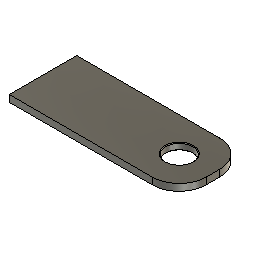
Lasche_19 (Autodesk Fusion 360 design; units mm, degrees)
Autodesk Fusion 360 part; units mm, degrees
sketch "Sketch1" plane through (0, 0, 0) normal (0, 0, 1) x (1, 0, 0)
  line L0 (-20.19, -5) -> (0, -5)
  line L1 (0, -5) -> (0, 5)
  line L2 (0, 5) -> (-20.19, 5)
  line L3 (-20.19, 5) -> (-20.19, -5)
  line L4 (0, 5) -> (1, 5)
  line L5 (5, 1) -> (5, -1)
  line L6 (1, -5) -> (0, -5)
  line L7 (0, -5) -> (0, 5)
  arc A0 (1, -5) -> (5, -1) centre (1, -1) ccw
  arc A1 (5, 1) -> (1, 5) centre (1, 1) ccw
  circle A2 centre (0, 0) radius 2
  point P0 (5, 5)
  dimension "d1" = 20.19
  dimension "d2" = 10
  dimension "d3" = 5
  dimension "d5" = 4
  dimension "d6" = 4
  dimension "d7" = 4
  constraint horizontal L0
  constraint vertical L1
  constraint horizontal L2
  constraint vertical L3
  constraint horizontal L4
  constraint vertical L5
  constraint horizontal L6
  constraint vertical L7
  constraint tangent L5 A0
  constraint tangent L6 A0
  constraint coincident P0 L4
  constraint coincident P0 L5
  constraint tangent L4 A1
  constraint tangent L5 A1
  constraint midpoint L1 A2.centre
  constraint coincident A2.centre origin
  measures "d1" distance of L0.start L0.end
  measures "d2" distance of L0.start L2.end
  measures "d3" distance of L1.end P0
  measures "d5" radius of A0
  measures "d6" radius of A1
  measures "d7" diameter of A2
extrude "Extrude1" add sketch "Sketch1" along normal mid plane 1 contours L0 L1 L2 L3 L7 A2 | L1 L4 L5 L6 L7 A0 A1 A2
chamfer "Chamfer1" distance 0.1 angle 45 2 edges at (-1.8647, 0.7232, 0.5) (-1.8647, -0.7232, -0.5)
